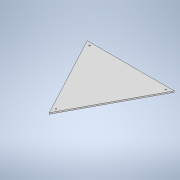
# Autodesk Inventor part: bcc_pcb
Saved by Autodesk Inventor 2020 (Build 240168000, 168)
## iProperties
Created: 2019-09-26
Part Number: bcc_pcb
Material: Generic
Document SubType Name: Modeling
Designer: fabrizio
Density: 1 g/cm^3
Appearance: Default
Author: fabrizio
Autodesk Inventor part; units mm, degrees
ref_plane "YZ Plane" through (0, 0, 0) normal (1, 0, 0) x (0, 1, 0)
ref_plane "XZ Plane" through (0, 0, 0) normal (0, 1, 0) x (-1, 0, 0)
ref_plane "XY Plane" through (0, 0, 0) normal (0, 0, 1) x (1, 0, 0)
sketch "Sketch1" plane through (0, 0, 0) normal (0, 1, 0) x (-1, 0, 0)
  line L0 (0, 0) -> (134.38, 0)
  line L1 (134.38, 0) -> (67.2135, 125.8908)
  line L2 (67.2135, 125.8908) -> (0, 0)
  circle A0 centre (8.2321, 4.6489) radius 1
  circle A1 centre (126.1421, 4.6489) radius 1
  circle A2 centre (67.2131, 115.5697) radius 1
  constraints: 6 end point, 3 centre point
extrude "Extrusion1" add sketch "Sketch1" along normal blind 2
body "Solid1"
